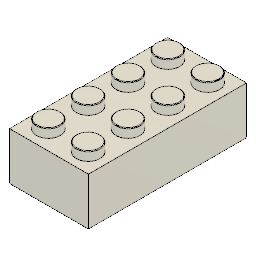
Lego Brick Reconstructed v1- DC-War-Story (Autodesk Fusion 360 design; units mm, degrees)
Autodesk Fusion 360 part; units mm, degrees
note: some values were not read from the file. Set by a fixed rule: which face or edge a step refers to.
sketch "Sketch1" plane through (0, 0, 0) normal (0, 1, 0) x (1, 0, 0)
  line L0 (7.938, 15.875) -> (-7.938, 15.875)
  line L1 (-7.938, 15.875) -> (-7.938, -15.875)
  line L2 (-7.938, -15.875) -> (7.938, -15.875)
  line L3 (7.938, -15.875) -> (7.938, 15.875)
  line L4 (7.938, 15.875) -> (-7.938, -15.875) construction
  line L5 (-7.938, 15.875) -> (7.938, -15.875) construction
  dimension "d1" = 15.876
  dimension "d2" = 31.75
  constraint horizontal L0
  constraint perpendicular L0 L1
  constraint parallel L0 L2
  constraint parallel L1 L3
  constraint coincident L4 origin
  constraint coincident L5 origin
  measures "d1" distance of L1.end L2.end
  measures "d2" distance of L0.end L1.end
extrude "Extrude1" add sketch "Sketch1" along normal blind 9.565
shell "Shell1" thickness 1.2 removed faces 1 at (2.646, 0, 5.2917)
sketch "Sketch2" plane through (0, 9.565, 0) normal (0, 1, 0) x (-1, 0, 0)
  line L0 (-7.938, 15.875) -> (-7.938, -15.875)
  line L1 (-7.938, -15.875) -> (7.938, -15.875)
  line L2 (7.938, -15.875) -> (7.938, 15.875)
  line L3 (7.938, 15.875) -> (-7.938, 15.875)
  line L4 (0, 0) -> (-4, 0) construction
  line L5 (-4, 0) -> (-4, -4) construction
  line L6 (-4, -4) -> (-4, -12) construction
  circle A0 centre (-4, -4) radius 2.4
  circle A1 centre (-4, -12) radius 2.4
  line L7 (0, 0) -> (0, -8) construction
  circle A2 centre (4, -12) radius 2.4
  circle A3 centre (4, -4) radius 2.4
  circle A4 centre (4, 4) radius 2.4
  circle A5 centre (4, 12) radius 2.4
  circle A6 centre (-4, 12) radius 2.4
  circle A7 centre (-4, 4) radius 2.4
  circle A8 centre (-4, -12) radius 1.2
  circle A9 centre (-4, -4) radius 1.2
  circle A10 centre (4, -12) radius 1.2
  circle A11 centre (4, -4) radius 1.2
  circle A12 centre (4, 12) radius 1.2
  circle A13 centre (-4, 12) radius 1.2
  circle A14 centre (-4, 4) radius 1.2
  circle A15 centre (4, 4) radius 1.2
  dimension "d6" = 4
  dimension "d7" = 4
  dimension "d8" = 8
  dimension "d9" = 4.8
  dimension "d10" = 4.8
  dimension "d11" = 8
  dimension "d14" = 2.4
  dimension "d15" = 2.4
  constraint coincident L4.start L7.start
  constraint horizontal L4
  constraint perpendicular L4 L5
  constraint parallel L5 L6
  constraint coincident L5.end L6.start
  constraint coincident L6.end A1.centre
  constraint perpendicular L4 L7
  constraint symmetric A0 L7 A3
  constraint symmetric A1 L7 A2
  constraint symmetric L4 A0 A7
  constraint symmetric L4 A1 A6
  constraint symmetric L4 A2 A5
  constraint symmetric L4 A3 A4
  constraint concentric A1 A8
  constraint concentric A0 A9
  constraint symmetric L7 A8 A10
  constraint symmetric L7 A9 A11
  constraint symmetric L4 A8 A13
  constraint symmetric L4 A9 A14
  constraint symmetric L4 A10 A12
  constraint symmetric L4 A11 A15
  measures "d6" distance of L4.start L4.end
  measures "d7" distance of L4.end L5.end
  measures "d8" distance of L5.end L6.end
  measures "d9" diameter of A0
  measures "d10" diameter of A1
  measures "d11" distance of L4.start L7.end
  measures "d14" diameter of A8
  measures "d15" diameter of A9
extrude "Extrude2" add sketch "Sketch2" along normal blind 1.8 contours A0 | A1 | A2 | A3 | A4 | A5 | A6 | A7 | A8 | A9 | A10 | A11 | A12 | A13 | A14 | A15
extrude "Extrude3" cut sketch "Sketch2" along normal blind 1.7 from surface at -1.2 contours A8 | A9 | A10 | A11 | A12 | A13 | A14 | A15
sketch "Sketch3" plane through (0, 8.365, 0) normal (0, -1, 0) x (1, 0, 0)
  circle A0 centre (4, 4) radius 1.2
  circle A1 centre (4, -12) radius 1.2
  circle A2 centre (-4, -4) radius 1.2
  circle A3 centre (-4, 12) radius 1.2
  circle A4 centre (-4, 4) radius 1.2
  circle A5 centre (-4, -12) radius 1.2
  circle A6 centre (4, -4) radius 1.2
  circle A7 centre (4, 12) radius 1.2
  line L0 (6.738, -14.675) -> (6.738, 14.675)
  line L1 (6.738, 14.675) -> (-6.738, 14.675)
  line L2 (-6.738, 14.675) -> (-6.738, -14.675)
  line L3 (-6.738, -14.675) -> (6.738, -14.675)
  line L4 (-4, 4) -> (4, 12) construction
  line L5 (-4, 12) -> (4, 4) construction
  line L6 (-4, -4) -> (4, -12) construction
  line L7 (4, -4) -> (-4, -12) construction
  circle A8 centre (0, 0) radius 3.255
  circle A9 centre (0, 8) radius 3.255
  circle A10 centre (0, -8) radius 3.255
  circle A11 centre (0, 0) radius 2.4
  circle A12 centre (0, 8) radius 2.4
  circle A13 centre (0, -8) radius 2.4
  dimension "d19" = 6.51
  dimension "d20" = 6.51
  dimension "d21" = 6.51
  dimension "d22" = 4.8
  dimension "d23" = 4.8
  dimension "d24" = 4.8
  constraint coincident A4.centre L4.start
  constraint coincident A7.centre L4.end
  constraint coincident A3.centre L5.start
  constraint coincident A0.centre L5.end
  constraint coincident A2.centre L6.start
  constraint coincident A1.centre L6.end
  constraint coincident A6.centre L7.start
  constraint coincident A5.centre L7.end
  constraint coincident A8.centre A11.centre
  constraint midpoint L5 A9.centre
  constraint midpoint L6 A10.centre
  constraint concentric A9 A12
  constraint concentric A10 A13
  measures "d19" diameter of A8
  measures "d20" diameter of A9
  measures "d21" diameter of A10
  measures "d22" diameter of A11
  measures "d23" diameter of A12
  measures "d24" diameter of A13
extrude "Extrude4" add sketch "Sketch3" along normal up to surface (8.365 mm away) contours A8 | A9 | A10
fillet "Fillet1" radius 0.12 8 edges at (-1.7624, 11.365, 3.1321) (-1.7624, 11.365, 11.1321) (6.2376, 11.365, 11.1321) (6.2376, 11.365, 3.1321) (-1.7624, 11.365, -4.8679) (6.2376, 11.365, -4.8679) (6.2376, 11.365, -12.8679) (-1.7624, 11.365, -12.8679)
equation "d20 = d19"
equation "d21 = d19"
equation "d23 = d22"
equation "d24 = d22"
